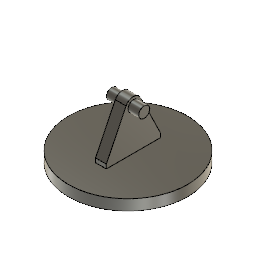
ENSAMB~2 (Autodesk Fusion 360 archive; units mm, degrees)
design "base_completa"
Autodesk Fusion 360 part; units mm, degrees
form "Forma1" [no effect]
sketch "Boceto4" plane through (0, 0, 0) normal (1, 0, 0) x (0, 1, 0)
  circle A0 centre (0, 38) radius 5
  line L0 (43.4267, 0) -> (42.975, 0)
  line L1 (-43.4267, 0) -> (-42.975, 0)
  line L2 (0, 0) -> (-25, 0)
  line L3 (-25, 0) -> (-25, 3.8109)
  line L4 (25, 0) -> (25, 3.8109)
  line L5 (0, 0) -> (25, 0)
  circle A1 centre (0, 38) radius 10
  line L6 (-25, 3.8109) -> (-9.2375, 41.8298)
  line L7 (25, 3.8109) -> (9.2375, 41.8298)
  point P0 (22.975, 0)
  point P1 (-22.975, 0)
  constraint horizontal L0
  constraint horizontal L1
  constraint coincident P1 L1
  constraint coincident P0 L0
  constraint coincident L2.start L5.start
  constraint perpendicular L2 L3
  constraint concentric A0 A1
  constraint coincident A1 L6.end
  constraint tangent A1 L6
  constraint coincident A1 L7.end
  constraint tangent A1 L7
sketch "Boceto8" plane through (0, 0, 0) normal (1, 0, 0) x (0, 1, 0)
  line L0 (-25, 0) -> (-25, 6)
  line L1 (465, 0) -> (465, 20)
  line L2 (-25, 6) -> (384.4, 6)
  line L3 (455, 30) -> (421, 30)
  line L4 (384.4, 6) -> (411, 6)
  line L5 (411, 6) -> (411, 20)
  arc A0 (465, 20) -> (455, 30) centre (455, 20) ccw
  arc A1 (421, 30) -> (411, 20) centre (421, 20) ccw
  line L6 (421, 30) -> (455, 30)
  line L7 (448, 0) -> (448, 24)
  line L8 (448, 24) -> (428, 24)
  line L9 (428, 24) -> (428, 0)
  line L10 (448, 0) -> (465, 0)
  line L11 (428, 0) -> (-25, 0)
  constraint vertical L0
  constraint vertical L1
  constraint perpendicular L0 L2
  constraint parallel L2 L4
  constraint perpendicular L4 L5
  constraint tangent L1 A0
  constraint tangent L5 A1
  constraint perpendicular L6 L7
  constraint perpendicular L8 L9
  constraint perpendicular L1 L10
  constraint perpendicular L0 L11
sketch "Boceto12" plane through (0, 0, 0) normal (1, 0, 0) x (0, 1, 0)
  line L0 (-43.4267, 10) -> (-42.975, 10)
  circle A0 centre (0, 48) radius 5
  line L1 (-25, 10) -> (-25, 13.8109)
  line L2 (43.4267, 10) -> (42.975, 10)
  line L3 (25, 10) -> (25, 13.8109)
  line L4 (55, 10) -> (55, 0)
  line L5 (55, 0) -> (-55, 0)
  line L6 (-55, 10) -> (-55, 0)
  line L7 (-55, 10) -> (55, 10)
  circle A1 centre (0, 48) radius 7.5
  line L8 (-25, 13.8109) -> (-6.7423, 51.2849)
  line L9 (25, 13.8109) -> (6.7423, 51.2849)
  point P0 (0, 10)
  point P1 (-22.975, 10)
  point P2 (22.975, 10)
  constraint horizontal L2
  constraint horizontal L0
  constraint coincident P1 L0
  constraint coincident P2 L2
  constraint perpendicular L4 L5
  constraint perpendicular L5 L6
  constraint perpendicular L4 L7
  constraint concentric A0 A1
  constraint coincident A1 L8.end
  constraint tangent A1 L8
  constraint coincident A1 L9.end
  constraint tangent A1 L9
extrude "Extruir13" add sketch "Boceto12" along normal mid plane 10 contours L1 L3 L7 A1 L8 L9 | A1 makes body 1
cylinder "CilindroPrimitivo3" add diameter 110 height 10 placed x (1, 0, 0) y (0, 1, 0) z (0, 0, 1) at (0, 0, 0) bodies 1
sketch "Boceto14" plane through (0, 0, 0) normal (0, 0, -1) x (1, 0, 0)
  circle A0 centre (0, 0) radius 55
sketch "Boceto15" plane through (0, 0, 0) normal (0, 0, -1) x (1, 0, 0)
  circle A0 centre (0, 0) radius 55
  line L0 (1.6583, 2.5) -> (1.4994, 8.0231)
  line L1 (-1.6583, 2.5) -> (-1.4994, 8.0231)
  arc A1 (1.4994, 8.0231) -> (-1.4994, 8.0231) centre (0, 7.98) ccw
  arc A2 (-1.6583, 2.5) -> (-1.6583, -2.5) centre (0, 0) ccw
  arc A3 (1.6583, -2.5) -> (1.6583, 2.5) centre (0, 0) ccw
  line L2 (1.6583, -2.5) -> (1.4994, -8.0231)
  line L3 (-1.6583, -2.5) -> (-1.4994, -8.0231)
  arc A4 (-1.4994, -8.0231) -> (1.4994, -8.0231) centre (0, -7.98) ccw
  constraint coincident A3.start A2
  constraint concentric A2 A3
  constraint tangent L1 A1
  constraint tangent L0 A1
  constraint tangent L3 A4
  constraint tangent L2 A4
extrude "Extruir14" cut sketch "Boceto15" against normal blind 3 contours L0 L1 A1 A2 A3 L2 L3 A4 bodies 1
copy_body "Cuerpo - > Comp.6" bodies 1 removing the originals makes body 2 in component "Component'"
sketch "Boceto16" plane through (5, 0, 0) normal (1, 0, 0) x (0, 1, 0)
  circle A0 centre (0, 48) radius 5
  line L0 (-25, 10) -> (25, 10)
  line L1 (25, 10) -> (25, 13.8109)
  line L2 (25, 13.8109) -> (6.7423, 51.2849)
  arc A1 (6.7423, 51.2849) -> (-6.7423, 51.2849) centre (0, 48) ccw
  line L3 (-6.7423, 51.2849) -> (-25, 13.8109)
  line L4 (-25, 13.8109) -> (-25, 10)
  circle A2 centre (0, 48) radius 5
  constraint concentric A0 A2
extrude "Extruir15" add sketch "Boceto16" along normal blind 10 separate body contours A0 A2 makes body 3
extrude "Extruir16" add 1 faces at (5, 1.0391, 50.7493) along direction (-1, 0, 0) blind 10 on bodies 3 bodies 3
extrude "Extruir17" add 1 faces at (-5, 1.0391, 50.7493) along direction (-1, 0, 0) blind 10 on bodies 3 bodies 3
copy_body "Cuerpo - > Comp.7" bodies 3 removing the originals makes body 4 in component "Component''"
extrude "Extruir10" [suppressed]
copy_body "Cuerpo - > Comp.4" [suppressed] in component "Component"
moveface "MoveFace1" [suppressed] in component "Component"
move_body "Desplazar1" [suppressed] in component "Component"
extrude "Extruir11" [suppressed]
component "Component'" placed x (1, 0, 0) y (0, 1, 0) z (0, 0, 1) at (0, 0, 0)
component "Component''" placed x (1, 0, 0) y (0, 1, 0) z (0, 0, 1) at (0, 0, 0)

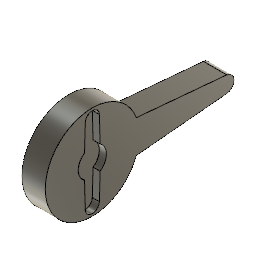
design "PinzaEscalada v1"
Autodesk Fusion 360 part; units mm, degrees
sketch "Boceto1" plane through (0, 0, 0) normal (1, 0, 0) x (0, 1, 0)
  arc A0 (85.8417, 2.5) -> (85.8417, -2.5) centre (87.5, 0) ccw
  arc A1 (89.1583, -2.5) -> (89.1583, 2.5) centre (87.5, 0) ccw
  line L0 (96.862, 3.505) -> (116.0692, 1.7779)
  line L1 (96.873, -3.4951) -> (116.0747, -1.7075)
  line L2 (85.8417, 2.5) -> (86.0006, 8.0231)
  line L3 (89.1583, 2.5) -> (88.9994, 8.0231)
  line L4 (85.8417, -2.5) -> (86.0006, -8.0231)
  line L5 (89.1583, -2.5) -> (88.9994, -8.0231)
  arc A2 (88.9994, 8.0231) -> (86.0006, 8.0231) centre (87.5, 7.98) ccw
  arc A3 (86.0006, -8.0231) -> (88.9994, -8.0231) centre (87.5, -7.98) ccw
  arc A4 (96.862, 3.505) -> (96.873, -3.4951) centre (87.5, -0.0098) ccw
  arc A5 (116.0747, -1.7075) -> (116.0692, 1.7779) centre (115.9125, 0.0349) ccw
  circle A6 centre (87.5, -0.0098) radius 2.5
  constraint coincident A1.start A0
  constraint concentric A0 A1
  constraint tangent L0 A5
  constraint tangent L1 A5
  constraint tangent L2 A2
  constraint tangent L3 A2
  constraint tangent L4 A3
  constraint tangent L5 A3
  constraint concentric A4 A6
extrude "Extruir5" add sketch "Boceto1" along normal blind 7 contours A0 A1 L2 L3 L4 L5 A2 A3 | A6 makes body 1
extrude "Extruir6" add sketch "Boceto1" along normal blind 10 contours L0 L1 A4 A5 bodies 1
sketch "Boceto2" plane through (0, 0, 0) normal (1, 0, 0) x (0, 1, 0)
extrude "Extruir7" add sketch "Boceto1" along normal blind 3.5 separate body contours A0 A1 L2 L3 L4 L5 A2 A3 | A6 makes body 2
extrude "Extruir8" add sketch "Boceto1" along normal blind 5 contours L0 L1 A4 A5 bodies 2
extrude "Extruir9" cut sketch "Boceto1" along normal blind 2.5 contours A6 bodies 2
scale "Escala1" factor 2 about (5, 96.862, 3.505) bodies 2
hidden bodies 1
